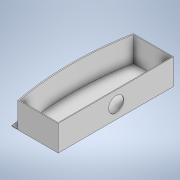
# Autodesk Inventor part: pièce_fixe_station
Saved by Autodesk Inventor 2020.2 (Build 242310000, 310)
## iProperties
Created: 2020-02-25
Part Number: pièce_fixe_station
Material: Générique
Document SubType Name: Modeling
Designer: anton
Density: 1 g/cm^3
Appearance: Par défaut
Author: anton
Autodesk Inventor part; units mm, degrees
ref_plane "YZ Plane" through (0, 0, 0) normal (1, 0, 0) x (0, 1, 0)
ref_plane "XZ Plane" through (0, 0, 0) normal (0, 1, 0) x (-1, 0, 0)
ref_plane "XY Plane" through (0, 0, 0) normal (0, 0, 1) x (1, 0, 0)
sketch "Esquisse1" plane through (0, 0, 0) normal (0, 1, 0) x (-1, 0, 0)
  arc A0 (8.3897, -168.8053) -> (8.3897, 132.3637) centre (-777.3166, -18.2208) ccw
  arc A1 (11.3897, -168.8053) -> (11.3897, 132.3637) centre (-774.3166, -18.2208) ccw
  line L0 (11.3897, 132.3637) -> (8.3897, 132.3637)
  line L1 (11.3897, -168.8053) -> (8.3897, -168.8053)
  point P0 (0, 0)
  dimension "d0" = 301.169
  constraints: 4 end point, 4 point on circle, 2 centre point, 1 parallel
  measures "d0" distance of L0.end L1.end
extrude "Extrusion1" add sketch "Esquisse1" along normal blind 65
sketch "Esquisse2" plane through (-11.3897, 0, 132.3637) normal (0, 0, 1) x (1, 0, 0)
  line L0 (0, 65) -> (3, 65) projected
  line L1 (0, 0) -> (3, 0) projected
  line L2 (0, 65) -> (3, 65)
  line L3 (3, 65) -> (3, 0)
  line L4 (3, 0) -> (0, 0)
  line L5 (0, 0) -> (0, 65)
  point P0 (11.3897, 0)
  constraints: 8 end point, 2 parallel, 1 horizontal, 1 perpendicular
extrude "Extrusion2" add sketch "Esquisse2" along normal blind 10
sketch "Esquisse3" plane through (-8.3897, 0, -168.8053) normal (0, 0, -1) x (-1, 0, 0)
  line L0 (0, 0) -> (3, 0) projected
  line L1 (3, 0) -> (3, 65) projected
  line L2 (0, 0) -> (3, 0)
  line L3 (3, 0) -> (3, 65)
  line L4 (3, 65) -> (0, 65)
  line L5 (0, 65) -> (0, 0)
  point P0 (-8.3897, 0)
  constraints: 8 end point, 2 parallel, 1 horizontal, 1 perpendicular
extrude "Extrusion3" add sketch "Esquisse3" along normal blind 10
sketch "Esquisse4" plane through (-8.3897, 0, 132.3637) normal (1, 0, 0) x (0, 0, -1)
  line L0 (0, 65) -> (-10, 65) projected
  line L1 (-10, 65) -> (-8, 65)
  line L2 (-8, 65) -> (-8, 0)
  line L3 (-8, 0) -> (-10, 0)
  line L4 (-10, 0) -> (-10, 65)
  line L5 (301.169, 0) -> (311.169, 0) projected
  line L6 (301.169, 65) -> (311.169, 65) projected
  line L7 (311.169, 0) -> (309.169, 0)
  line L8 (309.169, 0) -> (309.169, 65)
  line L9 (309.169, 65) -> (311.169, 65)
  line L10 (311.169, 65) -> (311.169, 0)
  point P0 (132.3637, 0)
  point P1 (309.169, 0)
  dimension "d10" = 2
  dimension "d11" = 2
  constraints: 16 end point, 4 parallel, 2 horizontal, 2 perpendicular, 1 point on line
  measures "d10" distance between parallel lines of L10 L8
  measures "d11" distance between parallel lines of L4 L2
extrude "Extrusion4" add sketch "Esquisse4" along normal blind 100
sketch "Esquisse5" plane through (0, 0, 0) normal (0, -1, 0) x (1, 0, 0)
  line L0 (91.6103, 140.3637) -> (91.6103, 142.3637) projected
  line L1 (-11.3897, 142.3637) -> (91.6103, 142.3637) projected
  line L2 (91.6103, 142.3637) -> (-11.3897, 142.3637)
  line L3 (-11.3897, 132.3637) -> (-11.3897, 142.3637) projected
  line L4 (-11.3897, 142.3637) -> (-11.3897, 132.3637)
  line L5 (91.6103, -176.8053) -> (91.6103, -178.8053) projected
  line L6 (91.6103, 142.3637) -> (91.6103, -178.8053)
  line L7 (-11.3897, -178.8053) -> (91.6103, -178.8053) projected
  line L8 (91.6103, -178.8053) -> (-11.3897, -178.8053)
  line L9 (-11.3897, -168.8053) -> (-11.3897, -178.8053) projected
  line L10 (-11.3897, -178.8053) -> (-11.3897, -168.8053)
  arc A0 (-11.3897, 132.3637) -> (-11.3897, -168.8053) centre (774.3166, -18.2208) ccw
  point P0 (0, 0)
  constraints: 10 end point, 2 collinear, 2 perpendicular, 2 point on circle, 1 centre point, 1 vertical
extrude "Extrusion5" add sketch "Esquisse5" along normal blind 2
sketch "Esquisse7" plane through (91.6103, 0, 132.3637) normal (1, 0, 0) x (0, 0, -1)
  line L0 (301.169, -2) -> (311.169, -2) projected
  line L1 (-10, 65) -> (311.169, 65)
  line L2 (311.169, 65) -> (311.169, -2)
  line L3 (311.169, -2) -> (-10, -2)
  line L4 (-10, -2) -> (-10, 65)
  point P0 (132.3637, 0)
  constraints: 8 end point, 2 parallel, 1 horizontal, 1 perpendicular
extrude "Extrusion6" add sketch "Esquisse7" along normal blind 2
sketch "Esquisse8" plane through (-11.3897, 65, -178.8053) normal (-1, 0, 0) x (0, 0, 1)
  line L0 (0, 0) -> (0, -67) projected
  line L1 (321.169, -67) -> (0, -67) projected
  line L2 (0, -65) -> (321.169, -65)
  line L3 (321.169, -65) -> (321.169, -67)
  line L4 (321.169, -67) -> (0, -67)
  line L5 (0, -67) -> (0, -65)
  point P0 (178.8053, -65)
  constraints: 8 end point, 2 parallel, 1 horizontal, 1 perpendicular, 1 point on line
extrude "Extrusion7" add sketch "Esquisse8" along normal blind 30
sketch "Esquisse9" plane through (-11.3897, 0, -168.8053) normal (0, 1, 0) x (1, 0, 0)
  arc A0 (0, 0) -> (0, -301.169) centre (785.7064, -150.5845) ccw projected
  line L0 (0, 0) -> (0, -301.169)
  line L1 (-30, -311.169) -> (-30, 10) projected
  arc A1 (-15.7, 0) -> (-15.7, -301.169) centre (770.0064, -150.5845) ccw
  line L2 (-15.7, 0) -> (0, 0)
  line L3 (-15.7, -301.169) -> (0, -301.169)
  line L4 (0, -301.169) -> (0, -311.169) projected
  arc A2 (0, 0) -> (0, -301.169) centre (785.7064, -150.5845) ccw
  line L5 (0, 0) -> (0, 10) projected
  line L6 (0, 0) -> (0, 10)
  line L7 (-30, 10) -> (-30, -311.169) projected
  line L8 (0, 10) -> (-30, 10)
  line L9 (-30, 10) -> (-30, -311.169)
  line L10 (0, -311.169) -> (-30, -311.169) projected
  line L11 (0, -311.169) -> (0, -301.169)
  point P0 (11.3897, -168.8053)
  point P1 (-30, -150.5845)
  constraints: 14 end point, 4 point on circle, 2 centre point, 2 parallel, 2 perpendicular, 2 vertical, 1 concentric, 1 horizontal
extrude "Extrusion8" cut sketch "Esquisse9" against normal through all contours L2 A1 L1 L8 L5 | L4 L10 L1 A1 L3
sketch "Esquisse10" plane through (93.6103, 0, 132.3637) normal (1, 0, 0) x (0, 0, -1)
  circle A0 centre (151.5428, 32.5) radius 20
  line L0 (311.169, 65) -> (-10, 65) projected
  point P0 (132.3637, 0)
  dimension "d36" = 40
  dimension "d37" = 32.5
  constraints: 1 centre point
  measures "d36" diameter of A0
  measures "d37" distance from line of L0 A0.centre
extrude "Extrusion9" cut sketch "Esquisse10" against normal blind 10
sketch "Esquisse11" plane through (-11.3897, 65, -178.8053) normal (-1, 0, 0) x (0, 0, 1)
  line L0 (10, -65) -> (10, 0) projected
  line L1 (10, 0) -> (-34.2459, 0)
  line L2 (-34.2459, 0) -> (-34.2459, -126.8111)
  line L3 (-34.2459, -126.8111) -> (10, -126.8111)
  line L4 (10, -126.8111) -> (10, 0)
  line L5 (311.169, -65) -> (311.169, 0) projected
  line L6 (311.169, 0) -> (416.0548, 0)
  line L7 (416.0548, 0) -> (416.0548, -178.3642)
  line L8 (416.0548, -178.3642) -> (311.169, -178.3642)
  line L9 (311.169, -178.3642) -> (311.169, 0)
  point P0 (178.8053, -65)
  constraints: 16 end point, 4 parallel, 2 horizontal, 2 perpendicular
extrude "Extrusion10" cut sketch "Esquisse11" against normal through all
sketch "Esquisse12" plane through (91.6103, 0, 132.3637) normal (-1, 0, 0) x (0, 0, 1)
  line L0 (-301.169, 0) -> (0, 0) projected
  line L1 (-301.169, 65) -> (0, 65) projected
  line L2 (-301.169, 0) -> (-299.169, 0)
  line L3 (-299.169, 0) -> (-299.169, 65)
  line L4 (-299.169, 65) -> (-301.169, 65)
  line L5 (-301.169, 65) -> (-301.169, 0)
  line L6 (0, 0) -> (-2, 0)
  line L7 (-2, 0) -> (-2, 65)
  line L8 (-2, 65) -> (0, 65)
  line L9 (0, 65) -> (0, 0)
  point P0 (-132.3637, 0)
  point P1 (-2, 0)
  dimension "d42" = 2
  dimension "d43" = 2
  constraints: 16 end point, 4 parallel, 2 horizontal, 2 perpendicular, 2 point on line
  measures "d42" distance between parallel lines of L5 L3
  measures "d43" distance between parallel lines of L9 L7
extrude "Extrusion11" add sketch "Esquisse12" along normal up to surface contours L5 L1 L3 L0 | L7 L1 L9 L0
